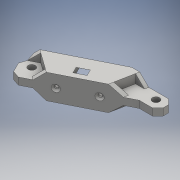
# Autodesk Inventor part: Support_GP2.Av
Saved by Autodesk Inventor 2016 (Build 200138000, 138)
## iProperties
Created: 2016-09-30
Part Number: Support_GP2.Av
Material: Générique
Document SubType Name: Modeling
Designer: LogOut
Density: 1 g/cm^3
Appearance: Par défaut
Author: LogOut
Autodesk Inventor part; units mm, degrees
ref_plane "YZ Plane" through (0, 0, 0) normal (1, 0, 0) x (0, 1, 0)
ref_plane "XZ Plane" through (0, 0, 0) normal (0, 1, 0) x (-1, 0, 0)
ref_plane "XY Plane" through (0, 0, 0) normal (0, 0, 1) x (1, 0, 0)
sketch "Esquisse1" plane through (0, 0, 0) normal (0, 0, 1) x (1, 0, 0)
  line L0 (156, 0) -> (156, 51.3475)
  line L1 (170, -60) -> (170, 60)
  line L2 (156, 0) -> (156, -52.5074)
  line L3 (-110, -100) -> (110, -100)
  line L4 (-78.695, 90) -> (-54, 90)
  line L5 (-156, 0) -> (-156, -52.5074)
  line L6 (-156, 0) -> (-156, 37.9311)
  line L7 (-170, 60) -> (-170, -60)
  line L8 (170, 60) -> (90, 100)
  line L9 (110, -100) -> (170, -60)
  line L10 (-170, -60) -> (-110, -100)
  line L11 (-90, 100) -> (-170, 60)
  line L12 (-156, 51.3475) -> (-78.695, 90)
  line L13 (-54, -90) -> (-54, 98)
  line L14 (-166, 57.5279) -> (-166, 0)
  line L15 (-166, 0) -> (-166, -52.5074)
  line L16 (-146, 31.3475) -> (-146, 0)
  line L17 (-146, 0) -> (-146, -52.5074)
  line L18 (-156, 51.3475) -> (-159.5777, 58.5029)
  line L19 (-156, 51.3475) -> (-150.6334, 40.6144)
  line L20 (-164, -52.5074) -> (-164, 0)
  line L21 (-164, 0) -> (-164, 56.2918)
  line L22 (-159.5777, 58.5029) -> (-80.5836, 98)
  line L23 (-80.5836, 98) -> (-54, 98)
  line L24 (-150.6334, 40.6144) -> (-75.8622, 78)
  line L25 (-75.8622, 78) -> (-54, 78)
  point P0 (54, -90)
  point P1 (-146, 42.9311)
  point P2 (-151.5279, 42.4033)
  dimension "d9" = 14
  dimension "d10" = 14
  dimension "d14" = 108
  dimension "d15" = 10
  dimension "d16" = 10
  dimension "d17" = 56
  dimension "d18" = 56
  dimension "d19" = 14
  dimension "d20" = 14
  dimension "d21" = 14
  constraints: 52 end point, 7 point on line, 4 vertical, 2 horizontal, 2 perpendicular, 1 parallel, 2 other
  measures "d9" distance from line of L7 L5.start
  measures "d10" distance from line of L1 L0.start
  measures "d14" distance of point (54, -90) L13.start
  measures "d15" distance from line of L3 point (54, -90)
  measures "d16" distance from line of L3 L13.start
  measures "d17" horizontal distance of L10.end L13.start
  measures "d18" horizontal distance of L9.start point (54, -90)
  measures "d19" distance from line of L8 L0.end
  measures "d20" distance from line of L9 L2.end
  measures "d21" distance from line of L10 L5.end
extrude "Extrusion1" add sketch "Esquisse1" along normal blind 28
move faces "Déplacer1" translate (-10.7331, -5.3666, 0) faces at (-158.3851, 56.1178, 9.3333) (-154.2111, 47.7698, 18.6667)
move faces "Déplacer2" translate (12, 0, 0) faces at (-54, 84.6667, 9.3333)
sketch "Esquisse18" plane through (0, 0, 28) normal (0, 0, 1) x (1, 0, 0)
  line L0 (-170, -60) -> (-110, -100)
  line L1 (-156, 0) -> (-156, -52.5074)
  line L2 (-156, 0) -> (-156, 37.9311)
  line L3 (-90, 100) -> (-170, 60)
  line L4 (-170, 60) -> (-170, -60)
  line L5 (156, 0) -> (156, 51.3475)
  line L6 (110, -100) -> (170, -60)
  line L7 (156, 0) -> (156, -52.5074)
  line L8 (170, -60) -> (170, 60)
  line L9 (170, 60) -> (90, 100)
  line L10 (-78.695, 90) -> (-54, 90)
  line L11 (-110, -100) -> (110, -100)
  line L12 (-156, 51.3475) -> (-78.695, 90)
  line L13 (-54, -90) -> (-54, 98)
  line L14 (-166, 57.5279) -> (-166, 0)
  line L15 (-166, 0) -> (-166, -52.5074)
  line L16 (-146, 31.3475) -> (-146, 0)
  line L17 (-146, 0) -> (-146, -52.5074)
  line L18 (-156, 51.3475) -> (-159.5777, 58.5029)
  line L19 (-156, 51.3475) -> (-150.6334, 40.6144)
  line L20 (-164, -52.5074) -> (-164, 0)
  line L21 (-164, 0) -> (-164, 56.2918)
  line L22 (-159.5777, 58.5029) -> (-80.5836, 98)
  line L23 (-80.5836, 98) -> (-54, 98)
  line L24 (-150.6334, 40.6144) -> (-75.8622, 78)
  line L25 (-75.8622, 78) -> (-54, 78)
  point P0 (0, 0)
  point P1 (54, -90)
  point P2 (-146, 42.9311)
  point P3 (-151.5279, 42.4033)
  dimension "d186" = 14
  dimension "d187" = 14
  dimension "d188" = 108
  dimension "d189" = 10
  dimension "d190" = 10
  dimension "d191" = 56
  dimension "d192" = 56
  dimension "d193" = 14
  dimension "d194" = 14
  dimension "d195" = 14
  constraints: 52 end point, 7 point on line, 4 vertical, 2 horizontal, 2 perpendicular, 1 parallel, 2 other
  measures "d186" distance from line of L4 L1.start
  measures "d187" distance from line of L8 L5.start
  measures "d188" distance of point (54, -90) L13.start
  measures "d189" distance from line of L11 point (54, -90)
  measures "d190" distance from line of L11 L13.start
  measures "d191" horizontal distance of L0.end L13.start
  measures "d192" horizontal distance of L6.start point (54, -90)
  measures "d193" distance from line of L9 L5.end
  measures "d194" distance from line of L6 L7.end
  measures "d195" distance from line of L0 L1.end
hole "Perçage5" at (-156, 51.3475, 28) at (-54, 90, 28) direction (0, 0, -1) diameter 8 end through all
move faces "Déplacer7" translate (1.7889, -3.5777, 0) faces at (-132.8651, 49.4986, 9.3333)
move faces "Déplacer8" translate (0, -6, 0) faces at (-58.612, 78, 18.6667)
move faces "Déplacer9" translate (-1.7889, 3.5777, 0) faces at (-140.4018, 68.0909, 18.6667)
sketch "Esquisse15" plane through (-172.0997, 56.7141, 28) normal (-0.4472136, 0.8944272, 0) x (0.8944272, 0.4472136, 0)
  line L0 (80.0902, 6) -> (32.0902, 6)
  line L1 (32.0902, 6) -> (32.0902, 22)
  line L2 (32.0902, 22) -> (80.0902, 22)
  line L3 (80.0902, 22) -> (80.0902, 6)
  line L4 (96.7902, 0) -> (0, 0)
  line L5 (96.7902, 28) -> (96.7902, 0)
  point P0 (128.5673, 28)
  point P1 (128.5673, 28)
  dimension "d166" = 48
  dimension "d167" = 16
  dimension "d168" = 6
  dimension "d169" = 16.7
  constraints: 12 end point, 2 parallel, 1 horizontal, 1 perpendicular
  measures "d166" distance between parallel lines of L3 L1
  measures "d167" distance between parallel lines of L2 L0
  measures "d168" distance between parallel lines of L4 L0
  measures "d169" distance between parallel lines of L5 L3
extrude "Extrusion8" cut sketch "Esquisse15" against normal blind 24
sketch "Esquisse16" plane through (-161.3666, 35.2478, 28) normal (-0.4472136, 0.8944272, 0) x (0.8944272, 0.4472136, 0)
  line L0 (74.5902, 14) -> (37.5902, 14)
  line L1 (80.0902, 22) -> (80.0902, 6)
  line L2 (32.0902, 22) -> (80.0902, 22)
  point P0 (128.5673, 28)
  point P1 (128.5673, 28)
  dimension "d172" = 37
  dimension "d173" = 5.5
  dimension "d174" = 8
  constraints: 6 end point, 1 horizontal
  measures "d172" distance of L0.start L0.end
  measures "d173" distance from line of L1 L0.start
  measures "d174" distance between parallel lines of L2 L0
hole "Perçage4" at (-94.651, 68.6056, 14) at (-127.7448, 52.0587, 14) direction (0.4472136, -0.8944272, 0) diameter 4 end through all
sketch "Esquisse17" plane through (-172.0997, 56.7141, 28) normal (-0.4472136, 0.8944272, 0) x (0.8944272, 0.4472136, 0)
  line L0 (96.7902, 6) -> (19.3902, 6)
  line L1 (19.3902, 6) -> (19.3902, 22)
  line L2 (19.3902, 22) -> (96.7902, 22)
  line L3 (96.7902, 22) -> (96.7902, 6)
  line L4 (80.0902, 6) -> (32.0902, 6)
  line L5 (32.0902, 22) -> (80.0902, 22)
  line L6 (96.7902, 28) -> (96.7902, 0)
  line L7 (80.0902, 22) -> (80.0902, 6)
  line L8 (32.0902, 6) -> (32.0902, 22)
  point P0 (128.5673, 28)
  point P1 (128.5673, 28)
  dimension "d182" = 16.7
  dimension "d183" = 12.7
  constraints: 18 end point, 3 collinear, 2 parallel, 1 horizontal, 1 perpendicular
  measures "d182" distance between parallel lines of L3 L7
  measures "d183" distance between parallel lines of L8 L1
extrude "Extrusion9" cut sketch "Esquisse17" against normal blind 24 contours L0 L7 L2 L3 | L0 L1 L2 L8
chamfer "Chanfrein10" distance 21.76 distance2 16.7 1 edges at (-74.7938, 78.532, 14) measured on face at (-75.0175, 78.9792, 14)
chamfer "Chanfrein11" distance 24 distance2 12.7 1 edges at (-144.0225, 43.9176, 14) measured on face at (-144.2461, 44.3648, 14)
sketch "Esquisse21" plane through (0, 0, 28) normal (0, 0, 1) x (1, 0, 0)
  line L0 (-154.7565, 65.3857) -> (-132.6642, 49.599) projected
  line L1 (-132.6642, 49.599) -> (-89.7317, 71.0653) projected
  line L2 (-89.7317, 71.0653) -> (-84.5261, 97.9965) projected
  line L3 (-84.5279, 98) -> (-84.5261, 97.9965) projected
  line L4 (-89.5279, 98) -> (-84.5279, 98) projected
  line L5 (-154.7565, 65.3857) -> (-89.5279, 98) projected
  line L6 (-80.3411, 98.5707) -> (-86.1787, 68.3696)
  line L7 (-86.1787, 68.3696) -> (-133.0299, 44.944)
  line L8 (-133.0299, 44.944) -> (-162.4863, 65.9929)
  line L9 (-162.4863, 65.9929) -> (-90.4721, 102)
  line L10 (-90.4721, 102) -> (-82.0557, 102)
  line L11 (-82.0557, 102) -> (-80.3411, 98.5707)
  line L12 (-162.4863, 65.9929) -> (-206.5562, 56.6568)
  line L13 (-206.5562, 56.6568) -> (-162.4863, 0)
  line L14 (-162.4863, 0) -> (-133.0299, 44.944)
  line L15 (-86.1787, 68.3696) -> (-30.292, 54.0182)
  line L16 (-30.292, 54.0182) -> (-36.7256, 118.0998)
  line L17 (-36.7256, 118.0998) -> (-80.3411, 98.5707)
  point P0 (0, 0)
  dimension "d216" = 4
  constraints: 24 end point, 5 other
  measures "d216" distance between parallel lines of L2 L6
extrude "Extrusion10" cut sketch "Esquisse21" against normal blind 10 contours L17 L16 L15 L6 | L14 L13 L12 L8
ref_plane "Plan de construction2" through (-89.5279, 98, 14) normal (0, 0, 1) x (1, 0, 0)
mirror "Symétrie1" about plane through (-89.5279, 98, 14) normal (0, 0, 1) of "Extrusion10"
move faces "Déplacer14" translate (0, 8, 0) faces at (-54.306, 72, 12.6667)
chamfer "Chanfrein12" distance 10 angle 45 4 edges at (-83.315, 83.1848, 18) (-83.315, 83.1848, 10) (-145.9171, 54.1529, 18) (-145.9171, 54.1529, 10)
sketch "Esquisse22" plane through (0, 0, 28) normal (0, 0, 1) x (1, 0, 0)
  line L0 (-74.9039, 74.007) -> (-70.2663, 98) projected
  line L1 (-70.2663, 98) -> (-80.4514, 98) projected
  line L2 (-86.1787, 68.3696) -> (-80.4514, 98) projected
  line L3 (-86.1787, 68.3696) -> (-74.9039, 74.007) projected
  arc A0 (-154.1954, 47.7777) -> (-159.9619, 51.8983) centre (-156, 51.3475) ccw projected
  line L4 (-154.1954, 47.7777) -> (-143.1492, 39.8844) projected
  line L5 (-143.1492, 39.8844) -> (-133.0299, 44.944) projected
  line L6 (-158.8043, 63.3618) -> (-133.0299, 44.944) projected
  line L7 (-158.8043, 63.3618) -> (-168.9236, 58.3021) projected
  line L8 (-168.9236, 58.3021) -> (-159.9619, 51.8983) projected
  line L9 (-81.2246, 94) -> (-71.0395, 94)
  line L10 (-74.5187, 76) -> (-79.8622, 76)
  line L11 (-79.8622, 76) -> (-85.2218, 73.3202)
  line L12 (-80.7119, 75.5752) -> (-80.6298, 76)
  line L13 (-136.7119, 47.5752) -> (-146.8313, 42.5155)
  line L14 (-165.2416, 55.671) -> (-155.1222, 60.7307)
  point P0 (0, 0)
  dimension "d223" = 4
  constraints: 12 end point, 10 point on line
  measures "d223" distance between parallel lines of L2 L12
extrude "Extrusion11" cut sketch "Esquisse22" against normal blind 10 contours L10 L11 L2 L9 L0 | A0 L8 L14 L6 L13 L4
mirror "Symétrie2" about plane through (-89.5279, 98, 14) normal (0, 0, 1) of "Extrusion11"
sketch "Esquisse8" plane through (0, 0, 28) normal (0, 0, 1) x (1, 0, 0)
  line L0 (-110.3035, 71.9597) -> (-121.0366, 66.5931)
  line L1 (-121.0366, 66.5931) -> (-117.4589, 59.4377)
  line L2 (-117.4589, 59.4377) -> (-106.7258, 64.8043)
  line L3 (-106.7258, 64.8043) -> (-110.3035, 71.9597)
  line L4 (-133.0299, 44.944) -> (-86.0737, 68.4221) projected
  line L5 (-132.6642, 49.599) -> (-89.7317, 71.0653) projected
  point P0 (0, 0)
  dimension "d107" = 6
  dimension "d108" = 8
  dimension "d109" = 12
  dimension "d110" = 18
  dimension "d111" = 18
  constraints: 8 end point, 3 parallel, 1 perpendicular
  measures "d107" distance between parallel lines of L4 L2
  measures "d108" distance between parallel lines of L2 L0
  measures "d109" distance between parallel lines of L3 L1
  measures "d110" distance from line of L5.start L1
  measures "d111" distance from line of L5.end L3
extrude "Extrusion6" cut sketch "Esquisse8" against normal blind 10
chamfer "Chanfrein7" distance 8 distance2 6 1 edges at (-115.6701, 69.2764, 22) measured on face at (-115.8937, 69.7236, 22)
chamfer "Chanfrein16" distance 2 angle 45 6 edges at (-122.1422, 81.6928, 22) (-87.0279, 98, 22) (-87.0279, 98, 6) (-122.1422, 81.6928, 6) (-125.956, 48.481, 12) (-92.8622, 65.0279, 12)
chamfer "Chanfrein17" distance 6 angle 45 3 edges at (-42, 98, 14) (-42, 80, 14) (-159.5777, 31.6701, 14)
ref_plane "Plan de construction4" through (-172.0997, 56.7141, 0) normal (-0.9486833, 0.3162278, 0) x (0, 0, 1)
sketch "Esquisse24" plane through (-172.0997, 56.7141, 0) normal (-0.9486833, 0.3162278, 0) x (0, 0, 1)
  line L0 (32.6031, 85.8887) -> (-4.0684, 85.8887)
  line L1 (-4.0684, 85.8887) -> (-4.0684, -31.594)
  line L2 (-4.0684, -31.594) -> (32.6031, -31.594)
  line L3 (32.6031, -31.594) -> (32.6031, 85.8887)
  point P0 (0, 0.619)
  constraints: 8 end point, 2 parallel, 1 horizontal, 1 perpendicular
extrude "Extrusion12" cut sketch "Esquisse24" against normal up to surface (6.836 mm away)
move faces "Déplacer15" translate (0, 3.5, 0) faces at (-78.0811, 76, 19.7488)
move faces "Déplacer16" translate (0, 3.5, 0) faces at (-78.0811, 76, 8.2512)
